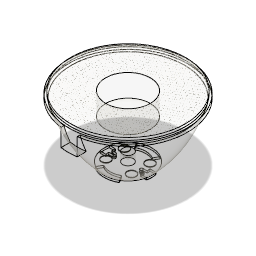
Zenka 2 degrees [MPLA000000111] v2 (Autodesk Fusion 360 design; units mm, degrees)
Autodesk Fusion 360 part; units mm, degrees
note: some values were not read from the file. Set by a fixed rule: which sketch regions a step uses.
sketch "Sketch1" plane through (0, 0, 0) normal (0, 0, 1) x (1, 0, 0)
  line L0 (15, 41.268) -> (15, 26.268)
  line L1 (0, 0) -> (0, 78.6649) construction
  arc A0 (15, 26.268) -> (0, 29.75) centre (0, -4.3) ccw
  line L2 (15, 41.268) -> (38.53, 41.268)
  line L3 (38.53, 41.268) -> (38.53, 39.568)
  line L4 (38.53, 39.568) -> (39.94, 39.568)
  line L5 (39.94, 39.568) -> (39.94, 37.018)
  line L6 (39.94, 37.018) -> (38.03, 37.018)
  line L7 (3.55, 0) -> (3.55, 6)
  line L8 (3.55, 0) -> (15.95, 0)
  arc A1 (15.95, 0) -> (38.03, 37.018) centre (-39.1763, 57.975) ccw
  arc A2 (0, 1) -> (3.55, 6) centre (-6.7538, 9.5555) ccw
  line L9 (0, 29.75) -> (0, 1)
  dimension "d7" = 15
  dimension "d8" = 15
  dimension "d9" = 34.05
  dimension "d10" = 4.3
  dimension "d11" = 38.53
  dimension "d12" = 1.7
  dimension "d13" = 1.41
  dimension "d14" = 2.55
  dimension "d15" = 1.91
  dimension "d16" = 6
  dimension "d18" = 3.55
  dimension "d19" = 15.95
  dimension "d20" = 80
  dimension "d22" = 10.9
  dimension "d23" = 1
  constraint vertical L0
  constraint coincident L1.start origin
  constraint vertical L1
  constraint coincident L1 A0.end
  constraint vertical L1.start A0.centre
  constraint perpendicular L0 L2
  constraint perpendicular L2 L3
  constraint perpendicular L1 L4
  constraint perpendicular L4 L5
  constraint perpendicular L5 L6
  constraint vertical L7
  constraint perpendicular L7 L8
  constraint coincident L1.start L8
  constraint coincident L1 A2.start
  measures "d7" distance of L0.start L0.end
  measures "d8" distance of L1.start L0
  measures "d9" radius of A0
  measures "d10" distance of L1.start A0.centre
  measures "d11" horizontal distance of L1.start L2.end
  measures "d12" distance of L2.end L3.end
  measures "d13" distance of L3.end L4.end
  measures "d14" distance of L4.end L5.end
  measures "d15" distance of L5.end L6.end
  measures "d16" distance of L7.start L7.end
  measures "d18" distance of L1.start L7
  measures "d19" horizontal distance of L1.start L8.end
  measures "d20" radius of A1
  measures "d22" radius of A2
  measures "d23" distance of L1.start A2.start
revolve "Revolve1" add sketch "Sketch1" angle 360 about axis through (0, 0, 0) along (0, 1, 0)
sketch "Sketch2" plane through (0, 0, 0) normal (0, -1, 0) x (1, 0, 0)
  circle A0 centre (0, 0) radius 15.95
  circle A1 centre (0, 0) radius 3.55
  line L0 (0, 15.95) -> (0, -15.95)
  line L1 (-15.95, 0) -> (15.95, 0)
  line L2 (-8, 15.95) -> (-8, -15.95)
  line L3 (8, 15.95) -> (8, -15.95)
  line L4 (-15.95, -3.15) -> (15.95, -3.15)
  line L5 (-15.95, 3.15) -> (15.95, 3.15)
  circle A2 centre (0, 0) radius 11.95
  circle A3 centre (0, 0) radius 8.125
  line L6 (8, 13.7986) -> (-8, -13.7986)
  line L7 (-8, 13.7986) -> (8, -13.7986)
  line L8 (-15.95, -1) -> (15.95, -1)
  line L9 (-15.95, 1) -> (15.95, 1)
  dimension "d25" = 8
  dimension "d26" = -8
  dimension "d27" = 3.15
  dimension "d28" = -3.15
  dimension "d29" = 23.9
  dimension "d30" = 16.25
  dimension "d33" = 1
  dimension "d34" = -1
  constraint coincident A0 L0.start
  constraint coincident A0 L0.end
  constraint vertical L0
  constraint coincident A0 L1.start
  constraint coincident A0 L1.end
  constraint perpendicular L0 L1
  constraint concentric A0 A2
  constraint concentric A2 A3
  constraint coincident L1 A0.centre
  constraint coincident L0 A0.centre
  constraint coincident L3 L6.start
  constraint coincident A0 L6.start
  constraint coincident L2 L6.end
  constraint coincident A0 L6.end
  constraint coincident L2 L7.start
  constraint coincident A0 L7.start
  constraint coincident L3 L7.end
  constraint coincident A0 L7.end
  measures "d29" diameter of A2
  measures "d30" diameter of A3
extrude "Extrude1" add sketch "Sketch2" along normal blind 1.31 contours A0 L0 A2 L6 | A0 L0 A2 L7 | A0 L5 A2 L9 | A0 L1 A2 L9 | A0 L5 A2 L9 | A0 L1 A2 L8 | L1 A2 A3 L9 | A0 L1 A2 L9 | A0 L4 A2 L8 | L1 A2 A3 L8 | L1 L3 A3 L9 | A0 L1 A2 L8 | L1 A2 A3 L9 | L1 L3 A3 L8 | A0 L4 A2 L8 | L1 A2 A3 L8 | L1 L2 A3 L9 | A0 L0 A2 L7 | L1 L2 A3 L8 | A0 L0 A2 L6
fillet "Fillet1" radius 1 4 edges at (-8, -0.655, 1) (-8, -0.655, -1) (8, -0.655, 1) (8, -0.655, -1)
sketch "Sketch3" plane through (0, -1.31, 0) normal (0, -1, 0) x (1, 0, 0)
  arc A0 (-9, -1) -> (-8, 0) centre (-9, 0) ccw
  arc A1 (-8, 0) -> (-9, 1) centre (-9, 0) ccw
  line L0 (-9, 1) -> (-11.9081, 1)
  arc A2 (-11.5274, 3.15) -> (-11.9081, 1) centre (0, 0) ccw
  line L1 (-11.5274, 3.15) -> (-15.6359, 3.15)
  arc A3 (-15.6359, 3.15) -> (-15.6359, -3.15) centre (0, 0) ccw
  line L2 (-15.6359, -3.15) -> (-11.5274, -3.15)
  arc A4 (-11.9081, -1) -> (-11.5274, -3.15) centre (0, 0) ccw
  line L3 (-11.9081, -1) -> (-9, -1)
  circle A5 centre (-9, 0) radius 0.885
  circle A6 centre (9, 0) radius 0.885
  arc A7 (8, 0) -> (9, -1) centre (9, 0) ccw
  dimension "d36" = 1.77
  dimension "d37" = 1.77
  constraint concentric A1 A5
  constraint concentric A6 A7
  measures "d36" diameter of A5
  measures "d37" diameter of A6
extrude "Extrude2" add sketch "Sketch3" along normal blind 0.9 contours A5 | A6
sketch "Sketch4" plane through (0, 0, 0) normal (0, -1, 0) x (1, 0, 0)
  line L0 (-11.5274, -3.15) -> (-15.6359, -3.15)
  arc A0 (-15.6359, -3.15) -> (-8, -13.7986) centre (0, 0) ccw
  line L1 (-8, -13.7986) -> (-5.9937, -10.3382)
  arc A1 (-5.9937, -10.3382) -> (5.9937, -10.3382) centre (0, 0) ccw
  line L2 (5.9937, -10.3382) -> (8, -13.7986)
  arc A2 (8, -13.7986) -> (15.6359, -3.15) centre (0, 0) ccw
  line L3 (15.6359, -3.15) -> (11.5274, -3.15)
  arc A3 (11.5274, -3.15) -> (11.9081, -1) centre (0, 0) ccw
  line L4 (11.9081, -1) -> (9, -1)
  arc A4 (8, 0) -> (9, -1) centre (9, 0) ccw
  arc A5 (9, 1) -> (8, 0) centre (9, 0) ccw
  line L5 (9, 1) -> (11.9081, 1)
  arc A6 (11.9081, 1) -> (11.5274, 3.15) centre (0, 0) ccw
  line L6 (11.5274, 3.15) -> (15.6359, 3.15)
  arc A7 (15.6359, 3.15) -> (8, 13.7986) centre (0, 0) ccw
  line L7 (8, 13.7986) -> (5.9937, 10.3382)
  arc A8 (5.9937, 10.3382) -> (-5.9937, 10.3382) centre (0, 0) ccw
  line L8 (-5.9937, 10.3382) -> (-8, 13.7986)
  arc A9 (-8, 13.7986) -> (-15.6359, 3.15) centre (0, 0) ccw
  line L9 (-15.6359, 3.15) -> (-11.5274, 3.15)
  arc A10 (-11.5274, 3.15) -> (-11.9081, 1) centre (0, 0) ccw
  line L10 (-11.9081, 1) -> (-9, 1)
  arc A11 (-8, 0) -> (-9, 1) centre (-9, 0) ccw
  arc A12 (-9, -1) -> (-8, 0) centre (-9, 0) ccw
  line L11 (-9, -1) -> (-11.9081, -1)
  arc A13 (-11.9081, -1) -> (-11.5274, -3.15) centre (0, 0) ccw
  circle A14 centre (0, 0) radius 3.55
  circle A15 centre (-8.6, 6.2) radius 3
  circle A16 centre (8.6, 6.2) radius 3
  circle A17 centre (8.6, -6.2) radius 3
  circle A18 centre (-8.6, -6.2) radius 3
  circle A19 centre (0, 0) radius 39.94
  circle A20 centre (0, 0) radius 33.54
  line L12 (0, 39.94) -> (0, 33.54)
  line L13 (-5.4, 39.5733) -> (-5.4, 33.1024)
  line L14 (5.4, 39.5733) -> (5.4, 33.1024)
  circle A21 centre (0, 0) radius 39.94
  dimension "d44" = 5.4
  dimension "d45" = 5.4
  dimension "d46" = 6
  dimension "d47" = 6
  dimension "d48" = 6
  dimension "d49" = 6
  dimension "d50" = 8.6
  dimension "d51" = 8.6
  dimension "d53" = 6.2
  dimension "d62" = 67.08
  dimension "d63" = 12.4
  constraint coincident A19 L12.start
  constraint coincident A20 L12.end
  constraint parallel L12 L14
  constraint coincident A20 L14.end
  constraint parallel L12 L13
  constraint coincident A20 L13.end
  constraint coincident A0.centre L12
  constraint coincident A19 L14.start
  constraint coincident A19 L13.start
  constraint vertical A15.centre A18.centre
  constraint horizontal A15.centre A16.centre
  constraint vertical A16.centre A17.centre
  constraint horizontal A17.centre A18.centre
  constraint coincident A0.centre A1.centre
  constraint vertical L12
  constraint concentric A19 A20
  measures "d44" distance of L12 L14
  measures "d45" distance of L12 L13
  measures "d46" diameter of A15
  measures "d47" diameter of A16
  measures "d48" diameter of A17
  measures "d49" diameter of A18
  measures "d50" horizontal distance of A15.centre A0.centre
  measures "d51" horizontal distance of A16.centre A0.centre
  measures "d53" vertical distance of A18.centre A0.centre
  measures "d62" diameter of A20
  measures "d63" distance of A16.centre A17.centre
extrude "Extrude3" cut sketch "Sketch4" against normal blind 0.35 contours A15 | A16 | A17 | A18
extrude "Extrude4" add sketch "Sketch4" along normal blind 11.8 from surface at -37.018 contours A19 A20 L12 L14 A21 | A19 A20 L12 L13 A21
sketch "Sketch8" plane through (0, -1.31, 0) normal (0, -1, 0) x (1, 0, 0)
  circle A0 centre (9, 0) radius 0.885
  arc A1 (8, 0) -> (9, -1) centre (9, 0) ccw
  line L0 (9, -1) -> (11.9081, -1)
  arc A2 (11.5274, -3.15) -> (11.9081, -1) centre (0, 0) ccw
  line L1 (11.5274, -3.15) -> (15.6359, -3.15)
  arc A3 (15.6359, -3.15) -> (15.6359, 3.15) centre (0, 0) ccw
  line L2 (15.6359, 3.15) -> (11.5274, 3.15)
  arc A4 (11.9081, 1) -> (11.5274, 3.15) centre (0, 0) ccw
  line L3 (11.9081, 1) -> (9, 1)
  arc A5 (9, 1) -> (8, 0) centre (9, 0) ccw
